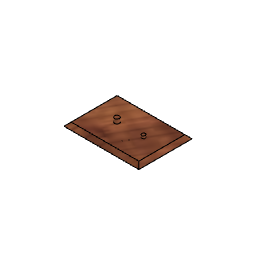
holder (Autodesk Fusion 360 design; units mm, degrees)
Autodesk Fusion 360 part; units mm, degrees
sketch "all" plane through (0, 0, 0) normal (0, 0, 1) x (1, 0, 0) in component "holder"
  circle A0 centre (-15, -0.0135) radius 19
  circle A1 centre (4, 10.9562) radius 7.95
  circle A2 centre (4, -0.0135) radius 2.1
  line L0 (-15, -0.0135) -> (4, -0.0135) construction
  line L1 (4, -0.0135) -> (4, 10.9562) construction
  circle A3 centre (4, 10.9562) radius 10.9697 construction
  line L2 (4, 10.9562) -> (-5.5, 5.4714) construction
  line L3 (4, 2.0865) -> (-6.9697, 2.0865)
  arc A4 (-6.9697, 2.0865) -> (-6.9697, -2.1134) centre (-6.9697, -0.0135) ccw
  line L4 (-6.9697, -2.1134) -> (4, -2.1134)
  arc A5 (4, -2.1134) -> (4, 2.0865) centre (4, -0.0135) ccw
  line L5 (4, -0.0135) -> (-6.9697, -0.0135) construction
  circle A6 centre (-15, 21.9258) radius 7.95
  line L6 (-9.1662, 5.891) -> (-3.6814, 15.391)
  arc A7 (-12.8035, 7.991) -> (-9.1662, 5.891) centre (-10.9848, 6.941) ccw
  line L7 (-7.3186, 17.491) -> (-12.8035, 7.991)
  arc A8 (-3.6814, 15.391) -> (-7.3186, 17.491) centre (-5.5, 16.441) ccw
  circle A9 centre (-34, 10.9562) radius 7.95
  line L8 (-17.1965, 7.991) -> (-22.6814, 17.491)
  arc A10 (-20.8338, 5.891) -> (-17.1965, 7.991) centre (-19.0152, 6.941) ccw
  line L9 (-26.3186, 15.391) -> (-20.8338, 5.891)
  arc A11 (-22.6814, 17.491) -> (-26.3186, 15.391) centre (-24.5, 16.441) ccw
  circle A12 centre (-34, -10.9831) radius 7.95
  line L10 (-23.0303, 2.0865) -> (-34, 2.0865)
  arc A13 (-23.0303, -2.1134) -> (-23.0303, 2.0865) centre (-23.0303, -0.0135) ccw
  line L11 (-34, -2.1134) -> (-23.0303, -2.1134)
  arc A14 (-34, 2.0865) -> (-34, -2.1134) centre (-34, -0.0135) ccw
  circle A15 centre (-15, -21.9528) radius 7.95
  line L12 (-20.8338, -5.918) -> (-26.3186, -15.418)
  arc A16 (-17.1965, -8.0179) -> (-20.8338, -5.918) centre (-19.0152, -6.968) ccw
  line L13 (-22.6814, -17.5179) -> (-17.1965, -8.0179)
  arc A17 (-26.3186, -15.418) -> (-22.6814, -17.5179) centre (-24.5, -16.468) ccw
  circle A18 centre (4, -10.9831) radius 7.95
  line L14 (-12.8035, -8.0179) -> (-7.3186, -17.5179)
  arc A19 (-9.1662, -5.918) -> (-12.8035, -8.0179) centre (-10.9848, -6.968) ccw
  line L15 (-3.6814, -15.418) -> (-9.1662, -5.918)
  arc A20 (-7.3186, -17.5179) -> (-3.6814, -15.418) centre (-5.5, -16.468) ccw
  circle A21 centre (-15, -0.0135) radius 2
  line L16 (14.8962, 17.5188) -> (14.5083, 17.2852)
  line L17 (-34, -10.9831) -> (-45, 8.0694)
  line L18 (-34, -10.9831) -> (-23, -30.0357)
  line L19 (-45, 8.0694) -> (2.6314, 35.5694)
  line L20 (-23, -30.0357) -> (24.6314, -2.5357)
  line L21 (26.3634, -1.5357) -> (24.6314, -2.5357)
  line L22 (4.3634, 36.5694) -> (2.6314, 35.5694)
  circle A22 centre (4, 10.9562) radius 1.5
  circle A23 centre (4, 10.9562) radius 14.7907
  line L23 (30.6936, 0.9643) -> (8.6936, 39.0694)
  line L24 (30.6936, 0.9643) -> (26.3634, -1.5357)
  line L25 (8.6936, 39.0694) -> (4.3634, 36.5694)
  line L26 (4, 10.9562) -> (0.025, 17.8411)
  line L27 (4, 10.9562) -> (7.975, 4.0713)
  line L28 (-0.75, 8.2138) -> (22.6021, 21.6961)
  circle A24 centre (15.673, 17.6956) radius 11.4075
  dimension "d3_1" = 38
  dimension "d8_1" = 360
  dimension "d9_1" = 4
  dimension "d10_1" = 15.9
  dimension "d11_1" = 22
  dimension "d12_1" = 22
  dimension "d13_1" = 55
  dimension "d14_1" = 55
  dimension "d15_1" = 55
  dimension "d17_1" = 3
  constraint coincident A0.centre L0.start
  constraint coincident A0 A2.centre
  constraint horizontal L0
  constraint coincident A2.centre L0.end
  constraint tangent A0 L1
  constraint perpendicular L0 L1
  constraint coincident A1.centre L1.end
  constraint concentric A1 A3
  constraint coincident A2.centre A3
  constraint coincident A0.centre L2
  constraint coincident A3 L2.end
  constraint tangent L3 A4
  constraint tangent A4 L4
  constraint parallel L3 L4
  constraint tangent L4 A5
  constraint tangent L3 A5
  constraint coincident L0 A4.centre
  constraint parallel L0 L5
  constraint equal A2 A5
  constraint equal L2 L5
  constraint coincident A3 A8.centre
  constraint concentric A0 A21
  constraint coincident A12.centre L17.start
  constraint perpendicular L17 L19
  constraint perpendicular L18 L20
  constraint concentric A1 A22
  constraint concentric A3 A23
  constraint coincident A1 L26.end
  constraint perpendicular L2 L26
  constraint coincident A1 L27.end
  constraint perpendicular L2 L27
  constraint midpoint L2 L28.start
  constraint perpendicular L23 L28
  constraint coincident L28 A24.centre
  measures "d3_1" diameter of A0
  measures "d9_1" diameter of A21
  measures "d10_1" diameter of A1
  measures "d11_1" distance of A12.centre L17.end
  measures "d12_1" distance of A12.centre L18.end
  measures "d13_1" distance of L17.end L19.end
  measures "d14_1" distance of L18.end L20.end
  measures "d15_1" distance of L18.end L20.end
  measures "d17_1" diameter of A22
extrude "Extrude1" add sketch "all" along normal blind 3 contours A0 A2 | A0 A2 A5 | A0 A2 L3 A4 L4 A23 | A0 A1 L3 A4 L6 A7 A23 | A0 A1 A2 L3 L4 A5 A18 A23 A24 | A0 L4 A18 A23 | A0 A1 | A0 A1 A22 L27 L28 | A0 A18 A23 | A0 A18 A23 | A0 A4 L4 A6 A7 L7 A9 L8 A10 L9 A12 L10 A13 L11 A15 L12 A16 L13 A18 L14 A19 L15 A23 | A4 L4 A23 | A0 A1 A22 L26 L28 | A0 A1 A6 L6 L7 A8 A23 A24 | A1 A22 L27 L28 A24 | A0 A18 L20 A23 | A0 A18 A23 | A18 L20 L21 A23 L23 L24 A24 | A22 L27 L28 | A22 L26 L28 | A0 L6 A7 L7 A23 | A0 L6 L7 A8 | A1 A22 L26 L28 A24 | A1 L28 A24 | A1 A23 L28 A24 | A22 L27 L28 | A7 L7 A23 | A0 A15 A18 L14 L15 A20 L20 | A23 L23 L28 A24 | A22 L26 L28 | A0 A6 L7 A23 | A1 A23 L28 A24 | A1 L28 A24 | A0 L14 L15 A20 | A0 L14 A19 L15 | A0 A6 A23 | A0 A6 A23 | A23 L23 L28 A24 | A6 L19 L22 A23 L23 L25 A24 | A0 A6 A23 | A0 A15 L20 | A0 A6 L19 A23 | A0 A6 A9 L8 L9 A11 L19 | A0 A15 | A0 A12 A15 L12 L13 A17 L18 L20 | A0 L8 A10 L9 | A0 L8 L9 A11 | A0 A9 L19 | A0 L12 L13 A17 | A0 L12 A16 L13 | A0 A12 L17 L18 | A0 A9 | A0 A9 A12 L10 L11 A14 L17 L19 | A0 A12 | A0 L10 A13 L11 | A0 L10 L11 A14 | A21 makes body 1 in component "holder"
extrude "Extrude2" add sketch "all" along normal blind 6 and the other way blind -4 separate body contours A0 A2 | A0 A2 A5 | A0 A2 L3 A4 L4 A23 | A0 A1 L3 A4 L6 A7 A23 | A0 A1 A2 L3 L4 A5 A18 A23 A24 | A0 L4 A18 A23 | A0 A1 | A0 A1 A22 L27 L28 | A0 A18 A23 | A0 A18 A23 | A0 A1 A22 L26 L28 | A0 A1 A6 L6 L7 A8 A23 A24 | A1 A22 L27 L28 A24 | A22 L27 L28 | A22 L26 L28 | A0 L6 A7 L7 A23 | A0 L6 L7 A8 | A1 A22 L26 L28 A24 | A1 L28 A24 | A1 A23 L28 A24 | A22 L27 L28 | A22 L26 L28 | A0 A6 L7 A23 | A1 A23 L28 A24 | A1 L28 A24 | A0 A6 A23 | A0 A6 A23 picked at (4.4049, -3.398) picked at (3.1093, -3.4881) picked at (-8.9544, 17.407) picked at (-8.2286, 18.4839) makes body 2 in component "holder"
extrude "Extrude3" add sketch "all" along normal blind 6 and the other way blind -7 contours A0 A1 | A0 A1 A22 L27 L28 | A0 A1 A22 L26 L28 | A1 A22 L27 L28 A24 | A22 L27 L28 | A22 L26 L28 | A1 A22 L26 L28 A24 | A1 L28 A24 | A22 L27 L28 | A22 L26 L28 | A1 L28 A24 bodies 2 in component "holder"
extrude "Extrude4" add sketch "all" along normal blind 10 and the other way blind -6 contours A0 A2 | A0 A2 L3 L4 A5 bodies 2 in component "holder"
delete_body "RemoveBody1" bodies 2 in component "holder"
extrude "Extrude5" add sketch "all" along normal blind 7 and the other way blind -6 separate body contours A0 A1 L3 A4 L6 A7 A23 | A0 L4 A18 A23 | A0 A4 L4 A6 A7 L7 A9 L8 A10 L9 A12 L10 A13 L11 A15 L12 A16 L13 A18 L14 A19 L15 A23 | A0 A6 L7 A23 | A21 makes body 3 in component "holder"
delete_body "RemoveBody2" bodies 3 in component "holder"
extrude "Extrude6" add sketch "all" along normal blind 6.5 contours A21 bodies 1 in component "holder"
extrude "Extrude7" add sketch "all" along normal blind 5 contours A22 L27 L28 | A22 L26 L28 | A22 L27 L28 | A22 L26 L28 bodies 1 in component "holder"
chamfer "Chamfer1" distance 3 angle 45 4 edges at (3.8468, -14.5357, 3) (19.6936, 20.0169, 3) (-18.1532, 23.5694, 3) (-34, -10.9831, 3) on bodies 1 in component "holder"
extrude "Extrude8" add sketch "all" along normal blind 7 and the other way blind -6 separate body contours A0 A1 | A0 A1 A22 L27 L28 | A0 A1 A22 L26 L28 | A1 A22 L27 L28 A24 | A22 L27 L28 | A22 L26 L28 | A1 A22 L26 L28 A24 | A22 L27 L28 | A22 L26 L28 makes body 4 in component "holder"
delete_body "RemoveBody3" bodies 4 in component "holder"
component "holder" placed x (1, 0, 0) y (0, 1, 0) z (0, 0, 1) at (0, 0, 0)
named bodies: "holder", "crank", "snowflake", "crank2"
